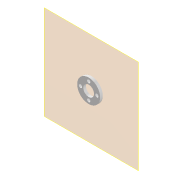
# Autodesk Inventor part: spool 4in inner plate
Saved by Autodesk Inventor 2020 (Build 240168000, 168)
## iProperties
Created: 2019-11-26
Part Number: spool 4in inner plate
Material: Generic
Document SubType Name: Modeling
Designer: ball
Density: 1 g/cm^3
Appearance: Default
Author: ball
Autodesk Inventor part; units mm, degrees
ref_plane "YZ Plane" through (0, 0, 0) normal (1, 0, 0) x (0, 1, 0)
ref_plane "XZ Plane" through (0, 0, 0) normal (0, 1, 0) x (-1, 0, 0)
ref_plane "XY Plane" through (0, 0, 0) normal (0, 0, 1) x (1, 0, 0)
ref_plane "Work Plane1" through (0, 0, 0) normal (0, 0, 1) x (1, 0, 0)
sketch "Sketch1" plane through (0, 0, 0) normal (0, 0, 1) x (1, 0, 0)
  arc A0 (-12.3389, 9.6089) -> (-9.6089, 12.3389) centre (-10.9739, 10.9739) ccw construction
  circle A1 centre (0, 9.779) radius 1.9304 projected
  circle A2 centre (9.6987, 0) radius 1.9304 projected
  circle A3 centre (0, -9.779) radius 1.9304 projected
  circle A4 centre (-9.779, 0) radius 1.9304 projected
  circle A5 centre (0, 0) radius 6.35 projected
  circle A6 centre (0, 0) radius 13.589
  constraints: 1 centre point, 1 coincident
extrude "Extrusion1" add sketch "Sketch1" along normal blind 3.175
body "Solid1"
